Autodesk Fusion 360 part; units mm, degrees
note: some values were not read from the file. Chosen so that the rebuilt part matches the saved one: which bodies a step acts on; which face or edge a step refers to; which pieces of a blend or face edit are solid. Set by a fixed rule: which sketch regions a step uses.
(part 2 of 2)
sketch "Skizze17" plane through (0, 0, 0) normal (-1, 0, 0) x (0, -1, 0)
  line L0 (6.3536, 1.4038) -> (4.9393, 2.818)
  line L1 (4.9393, 2.818) -> (9.182, 7.0607)
  line L2 (9.182, 7.0607) -> (10.5962, 5.6464)
  line L3 (10.5962, 5.6464) -> (11.3033, 6.3536)
  line L4 (11.3033, 6.3536) -> (16.9602, 0.6967)
  line L5 (16.9602, 0.6967) -> (18.1976, 1.9341)
  line L6 (18.1976, 1.9341) -> (19.9654, 0.1664)
  line L7 (19.9654, 0.1664) -> (18.3744, -1.4246)
  line L8 (18.3744, -1.4246) -> (19.0815, -2.1317)
  line L9 (19.0815, -2.1317) -> (22.6066, 1.3934)
  line L10 (22.6066, 1.3934) -> (12, 12)
  line L11 (12, 12) -> (12, 50)
  line L12 (12, 50) -> (0, 50)
  line L13 (0, 50) -> (0, 12)
  line L14 (0, 12) -> (-38, 12)
  line L15 (-38, 12) -> (-38, 0)
  line L16 (-38, 0) -> (0, 0)
  line L17 (0, 0) -> (10.6066, -10.6066)
  line L18 (10.6066, -10.6066) -> (14.1317, -7.0815)
  line L19 (14.1317, -7.0815) -> (13.4246, -6.3744)
  line L20 (13.4246, -6.3744) -> (11.8336, -7.9654)
  line L21 (11.8336, -7.9654) -> (10.0659, -6.1976)
  line L22 (10.0659, -6.1976) -> (11.3033, -4.9602)
  line L23 (11.3033, -4.9602) -> (5.6464, 0.6967)
  line L24 (5.6464, 0.6967) -> (6.3536, 1.4038)
  line L25 (6, 50) -> (6, 6) construction
  line L26 (-38, 6) -> (6, 6) construction
  line L27 (8, 5.8787) -> (6.1213, 4)
  line L28 (3.7574, 4) -> (-38, 4)
  line L29 (-38, 4) -> (-38, 8)
  line L30 (4, 50) -> (8, 50)
  line L31 (8, 50) -> (8, 8.2426)
  line L32 (-38, 8) -> (4, 8)
  line L33 (4, 8) -> (4, 50)
  line L34 (4.9393, 2.818) -> (3.7574, 4)
  line L35 (9.182, 7.0607) -> (8, 8.2426)
  line L36 (14.1317, 3.5251) -> (17.3033, 6.6967)
  line L37 (8.4749, -2.1317) -> (5.3033, -5.3033)
  circle A0 centre (15.7175, 5.1109) radius 1
  circle A1 centre (6.8891, -3.7175) radius 1
  line L38 (-38, 8) -> (4, 8)
  line L39 (2, 10) -> (-38, 10)
  line L40 (-38, 10) -> (-38, 8)
  line L41 (5.7574, 2) -> (-38, 2)
  line L42 (-38, 2) -> (-38, 4)
  line L43 (4, 50) -> (2, 50)
  line L44 (2, 50) -> (2, 10)
  line L45 (4, 10) -> (4, 50)
  line L46 (8, 50) -> (10, 50)
  line L47 (10, 50) -> (10, 6.2426)
  line L48 (4.9393, 2.818) -> (5.7574, 2)
  line L49 (9.182, 7.0607) -> (10, 6.2426)
  line L50 (-38, 4) -> (3.7574, 4)
  line L51 (8, 8.2426) -> (8, 50)
  circle A2 centre (-16.1213, 2) radius 1
  circle A3 centre (-16.1213, 2) radius 2
  line L52 (-16.1213, 2) -> (-16.1213, 10) construction
  circle A4 centre (-16.1213, 10) radius 2
  circle A5 centre (-16.1213, 10) radius 1
  circle A6 centre (10, 28.1213) radius 2
  circle A7 centre (10, 28.1213) radius 1
  line L53 (10, 28.1213) -> (2, 28.1213) construction
  circle A8 centre (2, 28.1213) radius 1
  circle A9 centre (2, 28.1213) radius 2
  line L54 (15.7175, 5.1109) -> (10, 10.8284)
  line L55 (15.7175, 5.1109) -> (18.5459, 2.2825)
  line L56 (18.5459, 2.2825) -> (18.1976, 1.9341)
  line L57 (6.8891, -3.7175) -> (1.1716, 2)
  line L58 (6.8891, -3.7175) -> (9.7175, -6.5459)
  line L59 (9.7175, -6.5459) -> (10.0659, -6.1976)
  circle A10 centre (15.7175, 5.1109) radius 2
  circle A11 centre (6.8891, -3.7175) radius 2
  dimension "d258" = 2
  dimension "d259" = 2
  dimension "d260" = 2
  dimension "d261" = 2
  dimension "d262" = 2
  dimension "d263" = 2
  dimension "d264" = 2
  dimension "d279" = 2
  dimension "d280" = 2
  dimension "d281" = 2
  dimension "d290" = 4
  dimension "d291" = 4
  constraint midpoint L15 L26.start
  constraint midpoint L12 L25.start
  constraint perpendicular L15 L26
  constraint coincident L1 L27.end
  constraint coincident L1 L27.start
  constraint horizontal L28
  constraint vertical L29
  constraint horizontal L32
  constraint horizontal L30
  constraint vertical L31
  constraint coincident L12 L30.start
  constraint coincident L0.end L1.start
  constraint perpendicular L1 L34
  constraint coincident L1.end L2.start
  constraint perpendicular L1 L35
  constraint midpoint L4 L36.start
  constraint midpoint L10 L36.end
  constraint midpoint L23 L37.start
  constraint midpoint L17 L37.end
  constraint midpoint L36 A0.centre
  constraint midpoint L37 A1.centre
  constraint horizontal L38
  constraint horizontal L39
  constraint vertical L40
  constraint horizontal L50
  constraint horizontal L41
  constraint vertical L42
  constraint horizontal L43
  constraint vertical L44
  constraint vertical L45
  constraint horizontal L46
  constraint vertical L47
  constraint coincident L0 L41.start
  constraint coincident L2 L47.end
  constraint midpoint L41 A2.centre
  constraint concentric A2 A3
  constraint tangent L50 A3
  constraint coincident A2.centre A3.centre
  constraint coincident L39 L52.end
  constraint perpendicular L39 L52
  constraint coincident L52.end A4.centre
  constraint tangent L38 A4
  constraint concentric A4 A5
  constraint midpoint L47 A6.centre
  constraint tangent L31 A6
  constraint concentric A6 A7
  constraint coincident A6.centre A7.centre
  constraint coincident L44 L53.end
  constraint perpendicular L44 L53
  constraint coincident L53.end A8.centre
  constraint concentric A8 A9
  constraint tangent L33 A9
  constraint tangent L45 A9
  constraint coincident A0.centre L54.start
  constraint coincident L47 L54.end
  constraint perpendicular L36 L54
  constraint perpendicular L5 L55
  constraint coincident L5.end L6.start
  constraint perpendicular L6 L56
  constraint coincident A1.centre L57.start
  constraint coincident L41 L57.end
  constraint perpendicular L37 L57
  constraint perpendicular L22 L58
  constraint coincident L21.end L22.start
  constraint perpendicular L21 L59
  constraint concentric A0 A10
  constraint concentric A1 A11
  measures "d258" diameter of A0
  measures "d259" diameter of A1
  measures "d260" distance of L29.end L39.end
  measures "d261" distance of L28.end L41.end
  measures "d262" distance of L30.start L43.end
  measures "d263" distance of L30.end L46.end
  measures "d264" diameter of A2
  measures "d279" diameter of A5
  measures "d280" diameter of A7
  measures "d281" diameter of A8
  measures "d290" diameter of A10
  measures "d291" diameter of A11
extrude "Extrusion72" cut sketch "Skizze17" against normal blind 2 contours L0 L23 L24 L37 L41 L57 A11 | L0 L28 L34 L41 L48 L50 A3 | L1 L12 L15 L27 L28 L29 L30 L31 L32 L33 L34 L35 L38 L45 L50 L51 | L16 L17 L37 L41 A3 L57 A11 | L22 L23 L37 L58 L59 A11 | L41 A2 A3 | L41 A2 A3 | L37 A1 L57 A11 | L37 A1 L57 A11 | L37 A1 L58 A11 | L15 L28 L41 L42 L50 A3 | L41 A2 | L41 A2 | L15 L16 L41 A3 | L37 A1 L57 | L37 A1 L57 | L17 L18 L19 L20 L21 L37 L58 L59 A11 | L37 A1 L58 A11 | L37 A1 L58 | L2 L31 L35 L47 L49 L51 A6 | L37 A1 L58 | L2 L3 L4 L36 L47 L54 A10 | L10 L11 L36 L47 A6 L54 A10 | L12 L31 L46 L47 L51 A6 | L47 A6 A7 | L47 A6 A7 | L36 A0 L54 A10 | L36 A0 L54 A10 | L11 L12 L47 A6 | L4 L5 L36 L55 L56 A10 | L47 A7 | L47 A7 | L36 A0 L54 | L36 A0 L54 | L36 A0 L55 A10 | L6 L7 L8 L9 L10 L36 L55 L56 A10 | L36 A0 L55 A10 | L36 A0 L55 | L36 A0 L55 bodies 5
extrude "Extrusion74" add 1 faces at (2, 25.3333, 12) along direction (0, 0, 1) blind 1 on bodies 5 bodies 5
extrude "Extrusion75" add 1 faces at (2, 0, 37.6667) along direction (0, 1, 0) blind 1 on bodies 5 bodies 5
extrude "Extrusion76" add 1 faces at (3.3333, 12.6667, 0) along direction (0, 0, -1) blind 1 on bodies 5 bodies 5
extrude "Extrusion77" add 1 faces at (4.6667, -7.0711, -7.0711) along direction (0, 0.707107, -0.707107) blind 1 on bodies 5 bodies 5
extrude "Extrusion78" add 1 faces at (4.6667, -12, 24.6667) along direction (0, -1, 0) blind 1 on bodies 5 bodies 5
extrude "Extrusion79" add 1 faces at (4.6667, -19.0711, 4.9289) along direction (0, -0.707107, 0.707107) blind 1 on bodies 5 bodies 5
extrude "Extrusion80" add sketch "Skizze17" against normal blind 2 contours L0 L28 L34 L41 L48 L50 A3 | L41 A2 A3 | L15 L28 L41 L42 L50 A3 | L2 L31 L35 L47 L49 L51 A6 | L12 L31 L46 L47 L51 A6 | L47 A6 A7 picked at (-16.2411, 3.6589) picked at (8.3411, 28.2411) bodies 5
extrude "Extrusion81" add 2 faces at (2, -14.167, 6.9006) (2, -5.0994, -2.167) along direction (-1, 0, 0) blind 2 on bodies 5 bodies 5
extrude "Extrusion82" add sketch "Skizze17" along normal blind 2 contours L0 L28 L34 L41 L48 L50 A3 | L41 A2 A3 | L41 A2 A3 | L15 L28 L41 L42 L50 A3 | L2 L31 L35 L47 L49 L51 A6 | L15 L32 L38 L39 L40 A4 | L12 L31 L46 L47 L51 A6 | L47 A6 A7 | L32 L33 L38 L39 L44 L45 A4 A9 | L39 A4 A5 | L47 A6 A7 | L39 A4 A5 | L12 L33 L43 L44 L45 A9 | L44 A8 A9 | L44 A8 A9 bodies 5
extrude "Extrusion83" cut sketch "Skizze17" against normal blind 6 contours L41 A2 | L41 A2 | L37 A1 L57 | L37 A1 L57 | L37 A1 L58 | L37 A1 L58 | L47 A7 | L47 A7 | L36 A0 L54 | L36 A0 L54 | L39 A5 | L39 A5 | L36 A0 L55 | L36 A0 L55 | L44 A8 | L44 A8 bodies 5
extrude "Extrusion84" add sketch "Skizze17" along normal blind 2 contours L0 L23 L24 L37 L41 L57 A11 | L22 L23 L37 L58 L59 A11 | L37 A1 L57 A11 | L37 A1 L57 A11 | L37 A1 L58 A11 | L37 A1 L58 A11 | L2 L3 L4 L36 L47 L54 A10 | L36 A0 L54 A10 | L36 A0 L54 A10 | L4 L5 L36 L55 L56 A10 | L36 A0 L55 A10 | L36 A0 L55 A10 bodies 5
copy_body "Körper kopieren/einfügen4" bodies 5 makes body 6
move_body "Verschieben14" bodies 6 to x (-1, 0, 0) y (0, 0, 1) z (0, 1, 0) at (-26.5, -12, 12)
move_body "Verschieben15" bodies 6 to x (1, 0, 0) y (0, 1, 0) z (0, 0, 1) at (26.5, 0, 0)
move_body "Verschieben16" bodies 6 to x (1, 0, 0) y (0, 1, 0) z (0, 0, 1) at (-16.5, 0, 0)
extrude "Extrusion85" cut 5 faces at (-14.5, 31.3738, 9.3333) (-14.5, -9.3333, 43.3738) (-14.5, 31.3738, 2.6667) (-14.5, -11.8689, 7.9024) (-14.5, -4.0976, 0.1311) along direction (-1, 0, 0) blind 4 on bodies 6 bodies 6
extrude "Extrusion86" cut 1 faces at (-17.1667, -10.1248, 6.1179) along direction (0, 0.707107, -0.707107) blind 6.5 on bodies 6 bodies 6
extrude "Extrusion87" cut 1 faces at (-17.1667, -13.1889, 4.4679) along direction (0, 0.707107, -0.707107) blind 8.5 on bodies 6 bodies 6
chamfer "Fase7" distance 2 angle 45 6 edges at (-22.5, 15.7597, 10.9323) (-22.5, 15.7597, 2.9323) (-22.5, -7.2507, -2.7852) (-22.5, -16.0791, 6.0432) (-22.5, -10.3616, 29.0536) (-22.5, -2.3616, 29.0536) on bodies 6
extrude "Extrusion88" cut 2 faces at (-21.1667, 38, 4.6667) (4.6667, 38, 5.3333) along direction (0, -1, 0) blind 18 on bodies 5 6 bodies 5 6
extrude "Extrusion89" cut 2 faces at (4.6667, -6.6667, 50) (-21.1667, -7.3333, 50) along direction (0, 0, -1) blind 18 on bodies 5 6 bodies 5 6
chamfer "Fase8" distance 0.5 angle 45 24 edges at (-2, 19.0607, 10) (-2, 16.1213, 12) (-2, 20, 9) (-2, 6.0607, 10) (-2, -2, 18.0607) (-2, 0, 28.1213) (-2, -2, 31.0607) (-2, -10, 31.0607) (-2, -12, 28.1213) (-2, -10, 18.4749) (-2, -12.1517, 8.6768) (-2, -17.1317, 6.5251) (-2, -17.8388, 2.9896) (-2, -17.753, 1.4896) (-2, -10.5104, -5.753) (-2, -9.0104, -5.8388) (-2, -5.4749, -5.1317) (-2, -3.3232, -0.1517) (-2, 6.4749, 2) (-2, 16.1213, 0) (-2, 19.0607, 2) (-2, 20, 3) (-2, -9, 32) (-2, -3, 32) on bodies 5
chamfer "Fase9" distance 0.5 angle 45 20 edges at (-16.5, -10, 31.0607) (-16.5, -12, 28.1213) (-16.5, -10, 18.4749) (-16.5, -12.1517, 8.6768) (-16.5, -17.1317, 6.5251) (-16.5, -17.8388, 2.9896) (-16.5, -2, 31.0607) (-16.5, -18.3718, 2.1083) (-16.5, 0, 28.1213) (-16.5, -2, 18.0607) (-16.5, 6.0607, 10) (-16.5, 16.1213, 12) (-16.5, 19.0607, 10) (-16.5, 19.0607, 2) (-16.5, 16.1213, 0) (-16.5, 6.4749, 2) (-16.5, -3.3232, -0.1517) (-16.5, -5.4749, -5.1317) (-16.5, -9.0104, -5.8388) (-16.5, -9.8917, -6.3718) on bodies 6
copy_body "Körper kopieren/einfügen5" bodies 5 makes body 7
move_body "Verschieben17" bodies 7 to x (1, 0, 0) y (0, 1, 0) z (0, 0, 1) at (-94, 0, 0)
copy_body "Körper kopieren/einfügen6" bodies 6 makes body 8
move_body "Verschieben18" bodies 8 to x (1, 0, 0) y (0, 1, 0) z (0, 0, 1) at (-96, 0, 0)
move_body "Verschieben19" bodies 7 to x (1, 0, 0) y (0, -1, 0) z (0, 0, -1) at (0, -46.6274, -22.6274)
move_body "Verschieben20" bodies 8 to x (1, 0, 0) y (0, -1, 0) z (0, 0, -1) at (0, -46.6274, -22.6274)
sketch "Skizze18" plane through (0, 0, 0) normal (1, 0, 0) x (0, 1, 0)
  line L0 (0, 0) -> (-30, 0)
  line L1 (-30, 0) -> (-30, -14)
  line L2 (-16, -14) -> (0, -14)
  line L3 (0, -14) -> (0, 0)
  line L4 (-30, 0) -> (-16, 0)
  line L5 (-16, -14) -> (-16, -30)
  line L6 (-16, -30) -> (-30, -30)
  line L7 (-30, -30) -> (-30, 0)
  line L8 (0, -7) -> (0, -5)
  line L9 (0, -7) -> (0, -9)
  line L10 (-23, -30) -> (-21, -30)
  line L11 (-23, -30) -> (-25, -30)
  line L12 (-21, -30) -> (-21, -14)
  line L13 (-25, -30) -> (-25, -14)
  line L14 (-16, -5) -> (0, -5)
  line L15 (-16, -9) -> (0, -9)
  arc A0 (-16, -9) -> (-21, -14) centre (-16, -14) ccw
  arc A1 (-16, -5) -> (-25, -14) centre (-16, -14) ccw
  line L16 (0, -5) -> (0, -3)
  line L17 (-25, -30) -> (-27, -30)
  line L18 (-21, -30) -> (-19, -30)
  line L19 (0, -9) -> (0, -11)
  line L20 (0, -11) -> (-16, -11)
  line L21 (-19, -14) -> (-19, -30)
  line L22 (-27, -30) -> (-27, -14)
  line L23 (-16, -3) -> (0, -3)
  arc A2 (-16, -11) -> (-19, -14) centre (-16, -14) ccw
  arc A3 (-16, -3) -> (-27, -14) centre (-16, -14) ccw
  circle A4 centre (-8, -11) radius 2
  circle A5 centre (-8, -11) radius 1
  circle A6 centre (-8, -3) radius 2
  circle A7 centre (-8, -3) radius 1
  circle A8 centre (-19, -22) radius 2
  circle A9 centre (-19, -22) radius 1
  circle A10 centre (-27, -22) radius 2
  circle A11 centre (-27, -22) radius 1
  circle A12 centre (-23.7782, -6.2218) radius 2
  circle A13 centre (-23.7782, -6.2218) radius 1
  dimension "d307" = 30
  dimension "d308" = 14
  dimension "d309" = 14
  dimension "d310" = 30
  dimension "d311" = 2
  dimension "d312" = 2
  dimension "d313" = 2
  dimension "d314" = 2
  dimension "d315" = 5
  dimension "d316" = 9
  dimension "d317" = 2
  dimension "d318" = 2
  dimension "d319" = 2
  dimension "d320" = 2
  dimension "d321" = 3
  dimension "d322" = 11
  dimension "d323" = 2
  dimension "d324" = 2
  dimension "d325" = 2
  dimension "d326" = 2
  dimension "d327" = 2
  constraint horizontal L0
  constraint vertical L1
  constraint horizontal L2
  constraint vertical L3
  constraint coincident L0.start L3.end
  constraint horizontal L4
  constraint vertical L5
  constraint horizontal L6
  constraint vertical L7
  constraint midpoint L3 L8.start
  constraint perpendicular L0 L8
  constraint parallel L3 L9
  constraint midpoint L6 L10.start
  constraint parallel L6 L10
  constraint parallel L6 L11
  constraint perpendicular L2 L12
  constraint perpendicular L11 L13
  constraint perpendicular L3 L14
  constraint perpendicular L3 L15
  constraint tangent L12 A0
  constraint tangent L15 A0
  constraint tangent L13 A1
  constraint tangent L14 A1
  constraint perpendicular L14 L16
  constraint perpendicular L13 L17
  constraint perpendicular L12 L18
  constraint perpendicular L15 L19
  constraint perpendicular L12 L20
  constraint perpendicular L6 L21
  constraint perpendicular L14 L22
  constraint perpendicular L3 L23
  constraint tangent L20 A2
  constraint tangent L21 A2
  constraint tangent L23 A3
  constraint tangent L22 A3
  constraint midpoint L20 A4.centre
  constraint tangent L15 A4
  constraint concentric A4 A5
  constraint midpoint L23 A6.centre
  constraint tangent L14 A6
  constraint concentric A6 A7
  constraint midpoint L21 A8.centre
  constraint tangent L12 A8
  constraint concentric A8 A9
  constraint midpoint L22 A10.centre
  constraint tangent L13 A10
  constraint concentric A10 A11
  constraint midpoint A3 A12.centre
  constraint tangent A1 A12
  constraint concentric A12 A13
  measures "d307" distance of L0.start L0.end
  measures "d308" distance of L0.start L2.end
  measures "d309" distance of L0.end L4.end
  measures "d310" distance of L0.end L6.end
  measures "d311" distance of L8.start L8.end
  measures "d312" distance of L8.start L9.end
  measures "d313" distance of L10.start L10.end
  measures "d314" distance of L10.start L11.end
  measures "d315" radius of A0
  measures "d316" radius of A1
  measures "d317" distance of L8.end L16.end
  measures "d318" distance of L11.end L17.end
  measures "d319" distance of L10.end L18.end
  measures "d320" distance of L9.end L19.end
  measures "d321" radius of A2
  measures "d322" radius of A3
  measures "d323" diameter of A5
  measures "d324" diameter of A7
  measures "d325" diameter of A9
  measures "d326" diameter of A11
  measures "d327" diameter of A13
extrude "Extrusion90" add sketch "Skizze18" along normal blind 6 separate body contours L0 L1 L3 L4 L6 L7 L22 L23 A3 A6 A10 A12 | L3 L14 L16 L23 A6 | L3 L6 L8 L9 L10 L11 L12 L13 L14 L15 A0 A1 | L23 A6 A7 | L23 A6 A7 | L14 A1 L23 A3 A6 A12 | L3 L15 L19 L20 A4 | L6 L13 L17 L22 A10 | L2 L3 L5 L6 L20 L21 A2 A4 A8 | L12 L15 A0 L20 L21 A2 A4 A8 | L20 A4 A5 | L13 A1 L22 A3 A10 A12 | A3 A12 A13 | A3 A12 A13 | L22 A10 A11 | L22 A10 A11 | L20 A4 A5 | L6 L12 L18 L21 A8 | L21 A8 A9 | L21 A8 A9 makes body 9
extrude "Extrusion91" cut sketch "Skizze18" along normal blind 2 contours L3 L6 L8 L9 L10 L11 L12 L13 L14 L15 A0 A1 bodies 9
extrude "Extrusion92" add sketch "Skizze18" against normal blind 2 contours L3 L14 L16 L23 A6 | L23 A6 A7 | L23 A6 A7 | L14 A1 L23 A3 A6 A12 | L3 L15 L19 L20 A4 | L6 L13 L17 L22 A10 | L12 L15 A0 L20 L21 A2 A4 A8 | L20 A4 A5 | L13 A1 L22 A3 A10 A12 | A3 A12 A13 | A3 A12 A13 | L22 A10 A11 | L22 A10 A11 | L20 A4 A5 | L6 L12 L18 L21 A8 | L21 A8 A9 | L21 A8 A9 bodies 9
extrude "Extrusion93" add sketch "Skizze18" against normal blind 6 separate body contours L0 L1 L3 L4 L6 L7 L22 L23 A3 A6 A10 A12 | L3 L14 L16 L23 A6 | L3 L6 L8 L9 L10 L11 L12 L13 L14 L15 A0 A1 | L23 A6 A7 | L23 A6 A7 | L14 A1 L23 A3 A6 A12 | L3 L15 L19 L20 A4 | L6 L13 L17 L22 A10 | L2 L3 L5 L6 L20 L21 A2 A4 A8 | L12 L15 A0 L20 L21 A2 A4 A8 | L20 A4 A5 | L13 A1 L22 A3 A10 A12 | A3 A12 A13 | A3 A12 A13 | L22 A10 A11 | L22 A10 A11 | L20 A4 A5 | L6 L12 L18 L21 A8 | L21 A8 A9 | L21 A8 A9 makes body 10
extrude "Extrusion94" cut sketch "Skizze18" against normal blind 2 contours L3 L14 L16 L23 A6 | L3 L6 L8 L9 L10 L11 L12 L13 L14 L15 A0 A1 | L23 A6 A7 | L23 A6 A7 | L14 A1 L23 A3 A6 A12 | L3 L15 L19 L20 A4 | L6 L13 L17 L22 A10 | L12 L15 A0 L20 L21 A2 A4 A8 | L20 A4 A5 | L13 A1 L22 A3 A10 A12 | A3 A12 A13 | A3 A12 A13 | L22 A10 A11 | L22 A10 A11 | L20 A4 A5 | L6 L12 L18 L21 A8 | L21 A8 A9 | L21 A8 A9 bodies 10
move_body "Verschieben21" bodies 10 to x (1, 0, 0) y (0, 1, 0) z (0, 0, 1) at (-4, 0, 0)
copy_body "Körper kopieren/einfügen7" bodies 9 makes body 11
move_body "Verschieben22" bodies 11 to x (1, 0, 0) y (0, 1, 0) z (0, 0, 1) at (0, -121, 0)
move_body "Verschieben24" bodies 11 to x (1, 0, 0) y (0, 1, 0) z (0, 0, 1) at (-94, 54.3726, -21.6274)
move_body "Verschieben25" bodies 11 to x (1, 0, 0) y (0, 1, 0) z (0, 0, 1) at (0, -20, 0)
chamfer "Fase10" distance 2 angle 45 5 edges at (-10, -8.9323, -3.3616) (-10, -8.9323, -11.3616) (-10, -24.7105, -6.5834) (-10, -27.9323, -22.3616) (-10, -19.9323, -22.3616) on bodies 10
copy_body "Körper kopieren/einfügen9" bodies 10 makes body 12
move_body "Verschieben26" bodies 12 to x (1, 0, 0) y (0, 1, 0) z (0, 0, 1) at (-108.5, -66.6274, -21.6274)
move_body "Verschieben27" bodies 12 to x (1, 0, 0) y (0, 1, 0) z (0, 0, 1) at (0, -20, 0)
delete_face "Fläche löschen3" 2 faces at (-95.6667, -66.4608, -25.4608) (-95.6667, -65.8345, -24.7941) on bodies 7
delete_face "Fläche löschen4" 1 faces at (-95.6667, -66.4608, -31.7941) on bodies 7
delete_face "Fläche löschen5" 1 faces at (-95.6667, -66.0012, -32.4608) on bodies 7
delete_face "Fläche löschen6" 1 faces at (-112.6667, -66.151, -32.9608) on bodies 8
delete_face "Fläche löschen7" 1 faces at (-112.6667, -66.151, -24.2941) on bodies 8
copy_body "Körper kopieren/einfügen10" bodies 1 makes body 13
move_body "Verschieben28" bodies 13 to x (1, 0, 0) y (0, 1, 0) z (0, 0, 1) at (0, 66, 0)
move_body "Verschieben29" bodies 13 to x (1, 0, 0) y (0, 1, 0) z (0, 0, 1) at (-104, -240.6274, -52.6274)
move_body "Verschieben30" bodies 13 to x (1, 0, 0) y (0, -1, 0) z (0, 0, -1) at (0, -251.2548, -131.2548)
delete_face "Fläche löschen8" 2 faces at (-95.6667, -96.5941, -69.4608) (-95.6667, -96.5941, -75.7941) on bodies 13
delete_face "Fläche löschen9" 2 faces at (-95.6667, -96.7608, -68.7941) (-95.6667, -96.7608, -76.4608) on bodies 13
extrude "Extrusion95" add 2 faces at (-94.6667, -96.4274, -69.9608) (-94.6667, -96.4274, -75.2941) along direction (0, 1, 0) blind 3 on bodies 13 bodies 13
split "Teilen1" by plane through (-94, -93.4274, -78.6274) normal (0, 1, 0) bodies 13 makes body 14 at (-88, -87.8274, -70.2941)
move_body "Verschieben31" bodies 14 to x (1, 0, 0) y (0, 1, 0) z (0, 0, 1) at (0, 5, 0)
delete_body "Körper entfernen1" bodies 13
copy_body "Körper kopieren/einfügen11" bodies 14 makes body 15
move_body "Verschieben32" bodies 15 to x (-1, 0, 0) y (0, 1, 0) z (0, 0, -1) at (-210, 0, -159.2548)
move_body "Verschieben33" bodies 15 to x (1, 0, 0) y (0, 1, 0) z (0, 0, 1) at (22, 0, 14)
move_body "Verschieben34" bodies 15 to x (1, 0, 0) y (0, 1, 0) z (0, 0, 1) at (-18.5, 0, 0)
copy_body "Körper kopieren/einfügen12" bodies 3 makes body 16
move_body "Verschieben35" bodies 16 to x (1, 0, 0) y (0, 1, 0) z (0, 0, 1) at (0, -115, 0)
split "Teilen2" by plane through (-40, -95.2, -4) normal (0, -1, 0) bodies 16 makes body 17 at (-34, -98.5657, -6.8994)
delete_body "Körper entfernen2" bodies 16
copy_body "Körper kopieren/einfügen13" bodies 4 makes body 18
move_body "Verschieben36" bodies 18 to x (1, 0, 0) y (0, 1, 0) z (0, 0, 1) at (0, -115, 0)
split "Teilen3" by plane through (-57, -95.2, -4) normal (0, 1, 0) bodies 18 makes body 19 at (-65, -72.5185, -7.2351)
delete_body "Körper entfernen3" bodies 19
move_body "Verschieben37" bodies 17 to x (1, 0, 0) y (0, 1, 0) z (0, 0, 1) at (-54, 43.3726, -66.6274)
move_body "Verschieben38" bodies 17 to x (1, 0, 0) y (0, 1, 0) z (0, 0, 1) at (0, 50, 0)
move_body "Verschieben39" bodies 18 to x (1, 0, 0) y (0, 1, 0) z (0, 0, 1) at (-53.5, 43.3726, -66.6274)
move_body "Verschieben40" bodies 18 to x (1, 0, 0) y (0, 1, 0) z (0, 0, 1) at (0, 50, 0)
copy_body "Körper kopieren/einfügen14" bodies 12 makes body 20
move_body "Verschieben41" bodies 20 to x (1, 0, 0) y (0, 0, 1) z (0, -1, 0) at (0, -168.2548, 37)
move_body "Verschieben42" bodies 20 to x (1, 0, 0) y (0, 1, 0) z (0, 0, 1) at (0, 28.2, 0)
copy_body "Körper kopieren/einfügen15" bodies 11 makes body 21
move_body "Verschieben43" bodies 21 to x (1, 0, 0) y (0, 0, 1) z (0, -1, 0) at (0, -168.2548, 65)
move_body "Verschieben44" bodies 21 to x (1, 0, 0) y (0, 1, 0) z (0, 0, 1) at (0, 28.2, -28)
extrude "Extrusion96" cut 1 faces at (-117.1667, -88.4274, -71.2941) along direction (0, -1, 0) blind 4 on bodies 20 bodies 20
extrude "Extrusion97" cut 1 faces at (-89.3333, -88.4274, -71.9608) along direction (0, -1, 0) blind 4 on bodies 21 bodies 21
move_body "Verschieben45" bodies 21 to x (1, 0, 0) y (0, 1, 0) z (0, 0, 1) at (0, 4, 0)
move_body "Verschieben46" bodies 20 to x (1, 0, 0) y (0, 1, 0) z (0, 0, 1) at (0, 4, 0)
move_body "Verschieben47" bodies 12 to x (1, 0, 0) y (0, 1, 0) z (0, 0, 1) at (0, 2.2, 30)
move_body "Verschieben48" bodies 11 to x (1, 0, 0) y (0, 1, 0) z (0, 0, 1) at (0, 2.2, 30)
copy_body "Körper kopieren/einfügen16" bodies 20 21 makes body 22 makes body 23
move_body "Verschieben49" bodies 22 23 to x (1, 0, 0) y (0, 0, 1) z (0, -1, 0) at (0, -40.0548, 34.8)
extrude "Extrusion98" cut 2 faces at (-89.3333, 9.5726, -71.9608) (-117.1667, 9.5726, -71.2941) along direction (0, 1, 0) blind 4 on bodies 22 23 bodies 22 23
move_body "Verschieben50" bodies 22 23 to x (1, 0, 0) y (0, 1, 0) z (0, 0, 1) at (0, -15.4, 0)
move_body "Verschieben51" bodies 7 8 to x (1, 0, 0) y (0, 1, 0) z (0, 0, 1) at (0, 57.8, 30)
delete_face "Fläche löschen10" 1 faces at (-88.4444, -12.5159, -70.067) on bodies 17
delete_face "Fläche löschen11" 1 faces at (-88.4444, -17.1547, -76.2485) on bodies 17
chamfer "Fase11" distance 2 angle 45 2 edges at (-118.5, -13.6951, -68.2658) (-118.5, -13.6951, -76.2658) on bodies 18
extrude "Extrusion73" [suppressed]
extrude "Extrusion70" [suppressed]
extrude "Extrusion68" [suppressed]
extrude "Extrusion66" [suppressed]
extrude "Extrusion46" [suppressed]
extrude "Extrusion45" [suppressed]
extrude "Extrusion35" [suppressed]
extrude "Extrusion24" [suppressed]
extrude "Extrusion20" [suppressed]
hidden bodies 1 2 3 4 5 6 9 10
equation "d225 = ( 11.5 / 2 ) * 1 mm"
named bodies: "Vorlage Laser Feder", "Vorlage Laser Nut", "Vorlage Sensor Feder", "Vorlage Sensor Nut", "Vorlage Anschluss Feder", "Anschluss Feder", "Vorlage Anschluss Nut", "Anschluss Feder (1)", "Anschluss Nut", "Anschluss Nut (1)", "Vorlage Ecke Feder", "Vorlage Ecke Nut", "Ecke Feder", "Ecke Nut", "Vorlage Laser Feder (1)", "Laser Feder", "Laser Feder (1)", "Vorlage Sensor Feder (1)", "Sensor Feder", "Sensor Nut", "Vorlage Sensor Nut (1) (1)", "Ecke Nut (1)", "Ecke Feder (1)", "Ecke Feder (1) (1)", "Ecke Nut (1) (1)"
